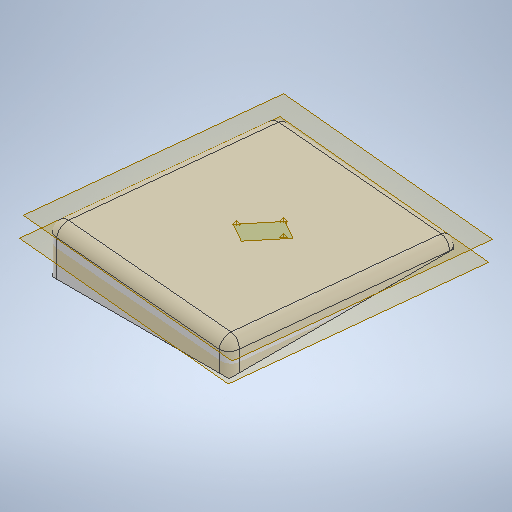
# Autodesk Inventor part: keycap
Saved by Autodesk Inventor 2025.2 (Build 292293000, 293)
## iProperties
Created: 2025-04-06
Part Number: keycap
Material: Generic
Document SubType Name: Modeling
Designer: nekita
Density: 1 g/cm^3
Appearance: Default
Author: nekita
Autodesk Inventor part; units mm, degrees
ref_plane "YZ Plane" through (0, 0, 0) normal (1, 0, 0) x (0, 1, 0)
ref_plane "XZ Plane" through (0, 0, 0) normal (0, 1, 0) x (-1, 0, 0)
ref_plane "XY Plane" through (0, 0, 0) normal (0, 0, 1) x (1, 0, 0)
sketch "Sketch1" plane through (0, 0, 0) normal (0, 1, 0) x (-1, 0, 0)
  line L0 (0, 0) -> (2.6246, 0) construction
  line L1 (0, 0) -> (0, -2.7039) construction
  line L2 (0, 0) -> (0, 2.7411) construction
  line L3 (0, 0) -> (-1.947, 0) construction
  line L4 (2, 0.64) -> (-2.4976, 0.64) construction
  line L5 (0.64, 2) -> (0.64, 0.64) construction
  line L6 (2, 0.64) -> (0.64, 0.64) construction
  line L7 (0.64, 2) -> (0.64, 0.64) construction
  line L8 (2, 0.64) -> (2, 0) construction
  line L9 (0.64, 2) -> (0, 2) construction
  line L10 (2, -0.64) -> (0.64, -0.64) construction
  line L11 (0.64, -2) -> (0.64, -0.64) construction
  line L12 (2, -0.64) -> (2, 0) construction
  line L13 (0.64, -2) -> (0, -2) construction
  line L14 (-2, 0.64) -> (-0.64, 0.64) construction
  line L15 (-0.64, 2) -> (-0.64, 0.64) construction
  line L16 (-2, 0.64) -> (-2, 0) construction
  line L17 (-0.64, 2) -> (0, 2) construction
  line L18 (-2, -0.64) -> (-0.64, -0.64) construction
  line L19 (-0.64, -2) -> (-0.64, -0.64) construction
  line L20 (-2, -0.64) -> (-2, 0) construction
  line L21 (-0.64, -2) -> (0, -2) construction
  line L22 (2.2, 0) -> (2.2, 0.84)
  line L23 (2.2, 0.84) -> (0.84, 0.84)
  line L24 (0.84, 0.84) -> (0.84, 2.2)
  line L25 (0.84, 2.2) -> (0, 2.2)
  line L26 (0, 2.2) -> (-0.84, 2.2)
  line L27 (-0.84, 2.2) -> (-0.84, 0.84)
  line L28 (-0.84, 0.84) -> (-2.2, 0.84)
  line L29 (-2.2, 0.84) -> (-2.2, 0)
  line L30 (-2.2, 0) -> (-2.2, -0.84)
  line L31 (-2.2, -0.84) -> (-0.84, -0.84)
  line L32 (-0.84, -0.84) -> (-0.84, -2.2)
  line L33 (-0.84, -2.2) -> (0, -2.2)
  line L34 (0, -2.2) -> (0.84, -2.2)
  line L35 (0.84, -2.2) -> (0.84, -0.84)
  line L36 (0.84, -0.84) -> (2.2, -0.84)
  line L37 (2.2, -0.84) -> (2.2, 0)
  circle A0 centre (0, 0) radius 2.8
  line L38 (-2.95, -2.95) -> (2.95, -2.95) construction
  line L39 (2.95, -2.95) -> (2.95, 2.95) construction
  line L40 (2.95, 2.95) -> (-2.95, 2.95) construction
  line L41 (-2.95, 2.95) -> (-2.95, -2.95) construction
  line L42 (-2.95, -2.95) -> (2.95, 2.95) construction
  line L43 (2.95, -2.95) -> (-2.95, 2.95) construction
  dimension "d0" = 4
  dimension "d1" = 1.28
  dimension "d2" = 0.2
  dimension "d3" = 5.6
  dimension "d6" = 5.9
  constraints: 88 end point, 11 symmetric about line, 7 perpendicular, 4 horizontal, 4 point on line, 3 equal length, 3 vertical, 2 midpoint, 1 centre point, 1 coincident, 15 other
  measures "d0" distance between parallel lines of L13 L9
  measures "d1" distance between parallel lines of L4 L10
  measures "d2" distance between parallel lines of L8 L22
  measures "d3" diameter of A0
  measures "d6" distance of L40.end L39.end
extrude "Extrusion1" add sketch "Sketch1" along normal blind 4
chamfer "Chamfer1" distance 0.2 angle 45 16 edges at (-0.84, 0, 1.52) (-0.42, 0, 2.2) (0.42, 0, 2.2) (0.84, 0, 1.52) (1.52, 0, 0.84) (2.2, 0, 0.42) (2.2, 0, -0.42) (1.52, 0, -0.84) (-1.52, 0, 0.84) (-2.2, 0, -0.42) (-2.2, 0, 0.42) (-1.52, 0, -0.84) (-0.84, 0, -1.52) (0.42, 0, -2.2) (-0.42, 0, -2.2) (0.84, 0, -1.52)
ref_plane "Work Plane1" through (-0.84, 4, 0.84) normal (0, 1, 0) x (1, 0, 0)
sketch "Sketch3" plane through (-0.84, 4, 0.84) normal (0, 1, 0) x (1, 0, 0)
  line L0 (9.96, 12.34) -> (-8.28, 12.34)
  line L1 (-8.28, 12.34) -> (-8.28, -10.66)
  line L2 (-8.28, -10.66) -> (9.96, -10.66)
  line L3 (9.96, -10.66) -> (9.96, 12.34)
  line L4 (9.96, 12.34) -> (-8.28, -10.66) construction
  line L5 (-8.28, 12.34) -> (9.96, -10.66) construction
  point P0 (0.84, 0.84)
  dimension "d11" = 23
  dimension "d12" = 18.24
  constraints: 12 end point, 2 midpoint, 2 parallel, 1 horizontal, 1 perpendicular
  measures "d11" distance of L0.end L1.end
  measures "d12" distance of L0.start L0.end
ref_plane "Work Plane2" through (-0.84, 7.4, 0.84) normal (0, 1, 0) x (1, 0, 0)
ref_plane "Work Plane5" through (-0.84, 6.95, 0.84) normal (0, 1, 0) x (1, 0, 0)
ref_plane "Work Plane6" through (-0.84, 7.4, 0.84) normal (-0.094484, -0.9910326, 0.094484) x (0.4796771, -0.1284849, -0.8679871)
extrude "Extrusion3" add sketch "Sketch3" along normal up to surface surface through (-0.84, 7.4, 0.84) normal (-0.094484, -0.9910326, 0.094484)
chamfer "Chamfer2" distance 0.4 angle 45 4 edges at (9.12, 4, 0) (0, 4, 11.5) (-9.12, 4, 0) (0, 4, -11.5)
ref_plane "Work Plane8" through (-9.309, 7.2237, 11.689) normal (0.094484, 0.9910326, -0.094484) x (0.9955264, -0.0940575, 0.0089673)
ref_plane "Work Plane7" through (-9.12, 9.2057, 11.5) normal (0.094484, 0.9910326, -0.094484) x (0.9955264, -0.0940575, 0.0089673)
sketch "Sketch4" plane through (-0.84, 0, 0.84) normal (0, -1, 0) x (1, 0, 0)
  line L0 (9.96, -12.34) -> (9.96, 10.66) projected
  line L1 (9.96, 10.66) -> (-8.28, 10.66) projected
  line L2 (-8.28, 10.66) -> (-8.28, -12.34) projected
  line L3 (-8.28, -12.34) -> (9.96, -12.34) projected
  line L4 (7.96, 8.66) -> (7.96, -10.34)
  line L5 (7.96, -10.34) -> (-6.28, -10.34)
  line L6 (-6.28, -10.34) -> (-6.28, 8.66)
  line L7 (-6.28, 8.66) -> (7.96, 8.66)
  circle A0 centre (0.84, -0.84) radius 2.8 projected
  circle A1 centre (0.84, -0.84) radius 2.8
  dimension "d24" = 2
  constraints: 8 end point, 1 centre point, 1 coincident, 1 concentric, 3 other
  measures "d24" distance between parallel lines of L0 L4
extrude "Extrusion4" cut sketch "Sketch4" against normal up to surface contours L4 L5 L6 L7 surface through (-9.309, 7.2237, 11.689) normal (0.094484, 0.9910326, -0.094484)
fillet "Fillet1" radius 1 8 edges at (9.12, 5.9334, 11.5) (9.12, 6.3703, 0) (0, 8.3362, 11.5) (9.12, 4.837, -11.5) (0, 6.1434, -11.5) (-9.12, 5.7065, -11.5) (-9.12, 8.1093, 0) (-9.12, 6.8029, 11.5)
ref_plane "Work Plane9" through (-0.84, 4.75, 0.84) normal (0, 1, 0) x (1, 0, 0)
sketch "Sketch6" plane through (-0.84, 4.75, 0.84) normal (0, 1, 0) x (1, 0, 0)
  line L0 (7.96, 6.5346) -> (4.1546, 10.34) projected
  line L1 (7.96, 6.5346) -> (7.96, -8.66) projected
  line L2 (7.96, -8.66) -> (-6.28, -8.66) projected
  line L3 (-6.28, -8.66) -> (-6.28, 10.34) projected
  line L4 (-6.28, 10.34) -> (4.1546, 10.34) projected
  circle A0 centre (0.84, 0.84) radius 2.8 projected
  line L5 (0.84, 0.84) -> (7.96, 0.84) construction
  line L6 (0.84, 0.84) -> (0.84, -8.66) construction
  line L7 (0.84, 0.84) -> (0.84, 10.34) construction
  line L8 (0.84, 0.84) -> (-6.28, 0.84) construction
  line L9 (7.96, 0.09) -> (3.5377, 0.09)
  line L10 (9.0545, 11.4345) -> (9.0545, -9.5655) projected
  circle A1 centre (0.84, 0.84) radius 2.8 projected
  line L11 (3.5377, 1.59) -> (7.96, 1.59)
  line L12 (7.96, 0.09) -> (7.96, 0.84)
  line L13 (7.96, 0.84) -> (7.96, 1.59)
  line L14 (1.59, 3.5377) -> (1.59, 10.34)
  line L15 (0.09, 3.5377) -> (0.09, 10.34)
  line L16 (1.59, 10.34) -> (0.84, 10.34)
  line L17 (0.09, 10.34) -> (0.84, 10.34)
  line L18 (1.59, -1.8577) -> (1.59, -8.66)
  line L19 (0.09, -1.8577) -> (0.09, -8.66)
  line L20 (-1.8577, 1.59) -> (-6.28, 1.59)
  line L21 (-1.8577, 0.09) -> (-6.28, 0.09)
  line L22 (1.59, -8.66) -> (0.09, -8.66)
  line L23 (-6.28, 1.59) -> (-6.28, 0.09)
  line L24 (-6.28, -8.66) -> (-6.28, 10.34) projected
  point P0 (-1.8577, 0.09)
  point P1 (0.09, -1.8577)
  point P2 (1.59, -1.8577)
  dimension "d29" = 1.5
  constraints: 36 end point, 11 point on line, 10 collinear, 9 perpendicular, 3 equal length, 2 midpoint, 10 other
  measures "d29" distance between parallel lines of L11 L9
extrude "Extrusion5" add sketch "Sketch6" along normal up to next contours L1 L9 A0 L11 | L14 A0 L15 L4 | A0 L21 L3 L20 | L2 L19 A0 L18
body "Solid1"
